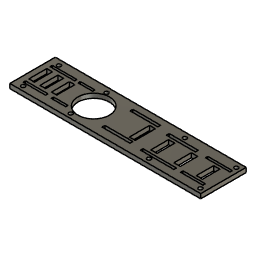
Drone Platform V9 - Secpnd Layer (Autodesk Fusion 360 design; units mm, degrees)
Autodesk Fusion 360 part; units mm, degrees
sketch "Sketch1" plane through (0, 0, 0) normal (0, 0, 1) x (1, 0, 0)
  line L0 (0, 40.6706) -> (170.6716, 40.6706)
  line L1 (170.6716, 40.6706) -> (170.6716, 0)
  line L2 (170.6716, 0) -> (0, 0)
  line L3 (0, 0) -> (0, 40.6706)
  constraint horizontal L0
  constraint vertical L1
  constraint horizontal L2
  constraint vertical L3
sketch "Sketch2" plane through (0, 0, 0) normal (0, 0, 1) x (1, 0, 0)
  circle A0 centre (2.5, 4) radius 1.75
  line L0 (170.6716, 0) -> (0, 0)
  line L1 (0, 0) -> (0, 40.6706)
  dimension "d1" = 3.5
  dimension "d2" = 4
  dimension "d3" = 2.5
  measures "d1" diameter of A0
  measures "d2" distance of A0.centre L0
  measures "d3" distance of A0.centre L1
sketch "Sketch4" plane through (0, 0, 0) normal (0, 0, 1) x (1, 0, 0)
  circle A0 centre (49.5, 4) radius 1.75
  circle A1 centre (2.5, 4) radius 1.75
  dimension "d9" = 3.5
  dimension "d10" = 47
  measures "d9" diameter of A0
  measures "d10" distance of A0.centre A1.centre
extrude "Extrude1" add sketch "Sketch1" along normal blind 4
sketch "Sketch11" plane through (0, 0, 4) normal (0, 0, 1) x (-1, 0, 0)
  line L0 (0, 0) -> (-170.6716, 0)
  line L1 (-170.6716, 0) -> (-170.6716, -40.6706)
  line L2 (-170.6716, -40.6706) -> (0, -40.6706)
  line L3 (0, -40.6706) -> (0, 0)
  line L4 (-5, -30) -> (-150, -30)
  line L5 (-150, -30) -> (-150, -10)
  line L6 (-150, -10) -> (-5, -10)
  line L7 (-5, -10) -> (-5, -30)
  constraint horizontal L4
  constraint vertical L5
  constraint horizontal L6
  constraint vertical L7
sketch "Sketch13" plane through (0, 0, 4) normal (0, 0, 1) x (-1, 0, 0)
  line L0 (0, 0) -> (-170.6716, 0)
  line L1 (-170.6716, 0) -> (-170.6716, -40.6706)
  line L2 (-170.6716, -40.6706) -> (0, -40.6706)
  line L3 (0, -40.6706) -> (0, 0)
  circle A0 centre (-8, -4) radius 1.75
  circle A1 centre (-8, -36) radius 1.75
  circle A2 centre (-50.5, -36) radius 1.75
  circle A3 centre (-50.5, -4) radius 1.75
  circle A4 centre (-120.5, -4) radius 1.75
  circle A5 centre (-120.5, -36) radius 1.75
  circle A6 centre (-166.5, -4) radius 1.75
  circle A7 centre (-166.5, -36) radius 1.75
  dimension "d44" = 3.5
  dimension "d45" = 4
  dimension "d46" = 3.5
  dimension "d47" = 32
  dimension "d48" = 8
  dimension "d49" = 8
  dimension "d50" = 3.5
  dimension "d52" = 3.5
  dimension "d53" = 4
  dimension "d55" = 32
  dimension "d56" = 3.5
  dimension "d58" = 4
  dimension "d59" = 3.5
  dimension "d60" = 32
  dimension "d62" = 3.5
  dimension "d63" = 46
  dimension "d64" = 4
  dimension "d65" = 3.5
  dimension "d66" = 46
  dimension "d67" = 32
  measures "d44" diameter of A0
  measures "d45" distance of L0 A0.centre
  measures "d46" diameter of A1
  measures "d47" vertical distance of A0.centre A1.centre
  measures "d48" distance of L3 A1.centre
  measures "d49" distance of L3 A0.centre
  measures "d50" diameter of A2
  measures "d52" diameter of A3
  measures "d53" distance of L0 A3.centre
  measures "d55" distance of A2.centre A3.centre
  measures "d56" diameter of A4
  measures "d58" distance of L0 A4.centre
  measures "d59" diameter of A5
  measures "d60" distance of A4.centre A5.centre
  measures "d62" diameter of A6
  measures "d63" distance of A4.centre A6.centre
  measures "d64" distance of L0 A6.centre
  measures "d65" diameter of A7
  measures "d66" horizontal distance of A5.centre A7.centre
  measures "d67" distance of A6.centre A7.centre
extrude "Extrude5" cut sketch "Sketch13" against normal blind 15 contours A0 | A1 | A2 | A3 | A4 | A5 | A6 | A7
sketch "Sketch16" plane through (0, 0, 4) normal (0, 0, 1) x (-1, 0, 0)
  circle A0 centre (-120.5, -36) radius 1.75
  circle A1 centre (-50.5, -36) radius 1.75
  circle A2 centre (-50.5, -4) radius 1.75
  circle A3 centre (-120.5, -4) radius 1.75
  circle A4 centre (-166.5, -36) radius 1.75
  circle A5 centre (-8, -36) radius 1.75
  circle A6 centre (-8, -4) radius 1.75
  circle A7 centre (-166.5, -4) radius 1.75
  line L0 (0, 0) -> (-170.6716, 0)
  line L1 (-170.6716, 0) -> (-170.6716, -40.6706)
  line L2 (-170.6716, -40.6706) -> (0, -40.6706)
  line L3 (0, -40.6706) -> (0, 0)
  line L4 (-5, -33) -> (-27, -33)
  line L5 (-27, -33) -> (-27, -31)
  line L6 (-27, -31) -> (-5, -31)
  line L7 (-5, -31) -> (-5, -33)
  line L8 (-5, -6.9037) -> (-25, -6.9037)
  line L9 (-25, -6.9037) -> (-25, -8.99)
  line L10 (-25, -8.99) -> (-5, -8.99)
  line L11 (-5, -8.99) -> (-5, -6.9037)
  line L12 (-5, -28.024) -> (-10, -28.024)
  line L13 (-10, -28.024) -> (-10, -12)
  line L14 (-10, -12) -> (-5, -12)
  line L15 (-5, -12) -> (-5, -28.024)
  line L16 (-15, -28) -> (-20, -28)
  line L17 (-20, -28) -> (-20, -12)
  line L18 (-20, -12) -> (-15, -12)
  line L19 (-15, -12) -> (-15, -28)
  line L20 (-25.2942, -28) -> (-30, -28)
  line L21 (-30, -28) -> (-30, -12)
  line L22 (-30, -12) -> (-25.2942, -12)
  line L23 (-25.2942, -12) -> (-25.2942, -28)
  line L24 (-30, -33) -> (-43, -33)
  line L25 (-43, -33) -> (-43, -31)
  line L26 (-43, -31) -> (-30, -31)
  line L27 (-30, -31) -> (-30, -33)
  line L28 (-30, -9) -> (-43, -9)
  line L29 (-43, -9) -> (-43, -7)
  line L30 (-43, -7) -> (-30, -7)
  line L31 (-30, -7) -> (-30, -9)
  circle A8 centre (-55, -20) radius 14.1421
  line L32 (-94.9908, -12) -> (-100.1485, -12)
  line L33 (-100.1485, -12) -> (-100.1485, -30)
  line L34 (-100.1485, -30) -> (-94.9908, -30)
  line L35 (-94.9908, -30) -> (-94.9908, -12)
  line L36 (-114.4734, -27.5201) -> (-119.9683, -27.5201)
  line L37 (-119.9683, -27.5201) -> (-119.9683, -11.6326)
  line L38 (-119.9683, -11.6326) -> (-114.4734, -11.6326)
  line L39 (-114.4734, -11.6326) -> (-114.4734, -27.5201)
  line L40 (-134.7975, -27.5201) -> (-140.4499, -27.5201)
  line L41 (-140.4499, -27.5201) -> (-140.4499, -12)
  line L42 (-140.4499, -12) -> (-134.7975, -12)
  line L43 (-134.7975, -12) -> (-134.7975, -27.5201)
  line L44 (-154.7885, -27.5201) -> (-160.2653, -27.5201)
  line L45 (-160.2653, -27.5201) -> (-160.2653, -12)
  line L46 (-160.2653, -12) -> (-154.7885, -12)
  line L47 (-154.7885, -12) -> (-154.7885, -27.5201)
  line L48 (-75, -10) -> (-100, -10)
  line L49 (-100, -10) -> (-100, -7.452)
  line L50 (-100, -7.452) -> (-75, -7.452)
  line L51 (-75, -7.452) -> (-75, -10)
  line L52 (-110, -8.9897) -> (-139.8992, -8.9897)
  line L53 (-139.8992, -8.9897) -> (-139.8992, -6.7652)
  line L54 (-139.8992, -6.7652) -> (-110, -6.7652)
  line L55 (-110, -6.7652) -> (-110, -8.9897)
  line L56 (-145, -9.7245) -> (-165.0971, -9.7245)
  line L57 (-165.0971, -9.7245) -> (-165.0971, -7.5785)
  line L58 (-165.0971, -7.5785) -> (-145, -7.5785)
  line L59 (-145, -7.5785) -> (-145, -9.7245)
  line L60 (-75, -35) -> (-99.8075, -35)
  line L61 (-99.8075, -35) -> (-99.8075, -32.5523)
  line L62 (-99.8075, -32.5523) -> (-75, -32.5523)
  line L63 (-75, -32.5523) -> (-75, -35)
  line L64 (-110, -32.4558) -> (-136, -32.4558)
  line L65 (-136, -32.4558) -> (-136, -29.8985)
  line L66 (-136, -29.8985) -> (-110, -29.8985)
  line L67 (-110, -29.8985) -> (-110, -32.4558)
  line L68 (-145, -31.9897) -> (-167, -31.9897)
  line L69 (-167, -31.9897) -> (-167, -29.9185)
  line L70 (-167, -29.9185) -> (-145, -29.9185)
  line L71 (-145, -29.9185) -> (-145, -31.9897)
  dimension "d78" = 22
  dimension "d79" = 3
  dimension "d81" = 13
  dimension "d82" = 13
  constraint horizontal L4
  constraint vertical L5
  constraint horizontal L6
  constraint vertical L7
  constraint horizontal L8
  constraint vertical L9
  constraint horizontal L10
  constraint vertical L11
  constraint horizontal L12
  constraint vertical L13
  constraint horizontal L14
  constraint vertical L15
  constraint horizontal L16
  constraint vertical L17
  constraint horizontal L18
  constraint vertical L19
  constraint horizontal L20
  constraint vertical L21
  constraint horizontal L22
  constraint vertical L23
  constraint horizontal L24
  constraint vertical L25
  constraint horizontal L26
  constraint vertical L27
  constraint horizontal L28
  constraint vertical L29
  constraint horizontal L30
  constraint vertical L31
  constraint horizontal L32
  constraint vertical L33
  constraint horizontal L34
  constraint vertical L35
  constraint horizontal L36
  constraint vertical L37
  constraint horizontal L38
  constraint vertical L39
  constraint horizontal L40
  constraint vertical L41
  constraint horizontal L42
  constraint vertical L43
  constraint horizontal L44
  constraint vertical L45
  constraint horizontal L46
  constraint vertical L47
  constraint horizontal L48
  constraint vertical L49
  constraint horizontal L50
  constraint vertical L51
  constraint horizontal L52
  constraint vertical L53
  constraint horizontal L54
  constraint vertical L55
  constraint horizontal L56
  constraint vertical L57
  constraint horizontal L58
  constraint vertical L59
  constraint horizontal L60
  constraint vertical L61
  constraint horizontal L62
  constraint vertical L63
  constraint horizontal L64
  constraint vertical L65
  constraint horizontal L66
  constraint vertical L67
  constraint horizontal L68
  constraint vertical L69
  constraint horizontal L70
  constraint vertical L71
  measures "d78" distance of L4.start L4.end
  measures "d79" distance of L5 L27
  measures "d81" distance of L24.start L24.end
  measures "d82" distance of L28.start L28.end
extrude "Extrude8" cut sketch "Sketch16" against normal blind 15 contours L4 L5 L6 L7 | L8 L9 L10 L11 | L12 L13 L14 L15 | L16 L17 L18 L19 | L20 L21 L22 L23 | L24 L25 L26 L27 | L28 L29 L30 L31 | A8 | L32 L33 L34 L35 | L36 L37 L38 L39 | L40 L41 L42 L43 | L44 L45 L46 L47 | L48 L49 L50 L51 | L52 L53 L54 L55 | L56 L57 L58 L59 | L60 L61 L62 L63 | L64 L65 L66 L67 | L68 L69 L70 L71
